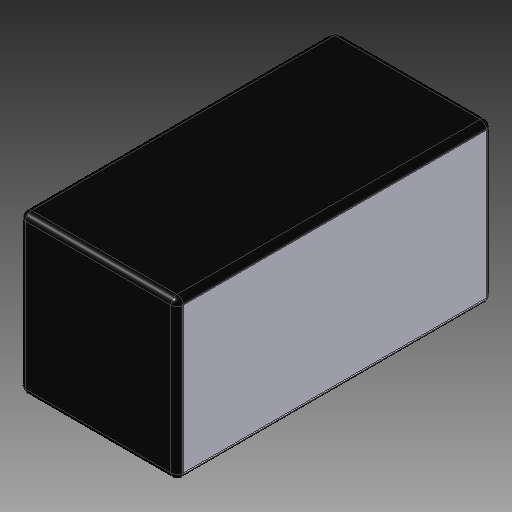
# Autodesk Inventor part: 1111A_Individual NdFeB Block_V1
Saved by Autodesk Inventor 2020 (Build 240168000, 168)
## iProperties
Created: 2019-10-13
Part Number: 1111A_Individual NdFeB Block_V1
Material: Stainless Steel
Document SubType Name: Modeling
Designer: RFLab
Density: 8 g/cm^3
Appearance: Semi-Polished
Mass: 2092.05 g
Surface Area: 251.042 cm^2
Volume: 261.506 cm^3
Author: RFLab
Autodesk Inventor part; units mm, degrees
ref_plane "YZ Plane" through (0, 0, 0) normal (1, 0, 0) x (0, 1, 0)
ref_plane "XZ Plane" through (0, 0, 0) normal (0, 1, 0) x (-1, 0, 0)
ref_plane "XY Plane" through (0, 0, 0) normal (0, 0, 1) x (1, 0, 0)
sketch "Sketch1" plane through (0, 0, 0) normal (0, 0, 1) x (1, 0, 0)
  line L0 (-25.4, -25.4) -> (25.4, -25.4)
  line L1 (25.4, -25.4) -> (25.4, 25.4)
  line L2 (25.4, 25.4) -> (-25.4, 25.4)
  line L3 (-25.4, 25.4) -> (-25.4, -25.4)
  line L4 (-25.4, -25.4) -> (25.4, 25.4) construction
  line L5 (25.4, -25.4) -> (-25.4, 25.4) construction
  point P0 (0, 0)
  dimension "d0" = 50.8
  dimension "d1" = 50.8
  constraints: 12 end point, 2 midpoint, 2 parallel, 1 horizontal, 1 perpendicular
  measures "d0" distance of L2.end L1.end
  measures "d1" distance of L1.end L0.end
extrude "Extrusion1" add sketch "Sketch1" along normal mid plane 101.6
fillet "Fillet1" radius 2 12 edges at (0, 25.4, 50.8) (-25.4, 25.4, 0) (-25.4, 0, 50.8) (-25.4, -25.4, 0) (0, -25.4, 50.8) (25.4, -25.4, 0) (25.4, 0, 50.8) (25.4, 25.4, 0) (-25.4, 0, -50.8) (0, -25.4, -50.8) (25.4, 0, -50.8) (0, 25.4, -50.8)
body "Solid1"
